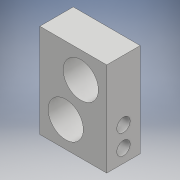
# Autodesk Inventor part: Part2
Saved by Autodesk Inventor 2017 (Build 210142000, 142)
## iProperties
Created: 2021-05-13
Part Number: Part2
Material: Generic
Document SubType Name: Modeling
Designer: majch
Density: 1 g/cm^3
Appearance: Default
Author: majch
Autodesk Inventor part; units mm, degrees
ref_plane "YZ Plane" through (0, 0, 0) normal (1, 0, 0) x (0, 1, 0)
ref_plane "XZ Plane" through (0, 0, 0) normal (0, 1, 0) x (-1, 0, 0)
ref_plane "XY Plane" through (0, 0, 0) normal (0, 0, 1) x (1, 0, 0)
sketch "Sketch1" plane through (0, 0, 0) normal (0, 1, 0) x (-1, 0, 0)
  line L0 (30, 18.75) -> (-10, 18.75)
  line L1 (30, 18.75) -> (30, -37.25)
  line L2 (-10, 18.75) -> (-10, -37.25)
  line L3 (-10, -37.25) -> (30, -37.25)
  circle A0 centre (5.5, 3.25) radius 10.5
  circle A1 centre (14.5, -21.75) radius 10.5
  point P0 (0, 0)
  dimension "szerokosc_jakas" = 40
  dimension "dlugosc_docisku" = 56
  dimension "srendica_walka" = 21
  dimension "odsuniecie_walka" = 15.5
  dimension "d4" = 15.5
  dimension "d5" = 21
  dimension "przesuniecie_wzgledne_walkow" = 9
  dimension "d7" = 25
  constraints: 8 end point, 2 centre point, 2 perpendicular, 1 horizontal
  measures "szerokosc_jakas" distance of L0.start L0.end
  measures "dlugosc_docisku" distance of L0.start L1.end
  measures "srendica_walka" diameter of A0
  measures "odsuniecie_walka" distance from line of L0 A0.centre
  measures "d4" distance from line of L2 A0.centre
  measures "d5" diameter of A1
  measures "przesuniecie_wzgledne_walkow" horizontal distance of A0.centre A1.centre
  measures "d7" vertical distance of A0.centre A1.centre
extrude "Extrusion1" add sketch "Sketch1" along normal blind 20
sketch "Sketch2" plane through (10, 0, 18.75) normal (1, 0, 0) x (0, 0, -1)
  circle A0 centre (48, 10) radius 4
  line L0 (56, 0) -> (56, 20) projected
  line L1 (0, 20) -> (56, 20) construction
  circle A1 centre (36, 10) radius 4
  line L2 (69, 10) -> (-3, 10) construction
  point P0 (18.75, 0)
  dimension "d10" = 8
  dimension "d11" = 8
  dimension "d15" = 12
  dimension "d25" = 10
  constraints: 2 centre point, 2 end point, 2 point on line, 1 horizontal
  measures "d10" diameter of A0
  measures "d11" distance from line of L0 A0.centre
  measures "d15" distance of A1.centre A0.centre
  measures "d25" distance between parallel lines of L1 L2
extrude "Extrusion2" cut sketch "Sketch2" against normal blind 10
sketch "Sketch3" plane through (-30, 0, -37.25) normal (-1, 0, 0) x (0, 0, 1)
  circle A0 centre (48, 10) radius 4
  circle A1 centre (36, 10) radius 4
  line L0 (56, 0) -> (56, 20) projected
  line L1 (0, 0) -> (56, 0) projected
  line L2 (75, 10) -> (-12, 10) construction
  point P0 (37.25, 0)
  dimension "d18" = 8
  dimension "d19" = 8
  dimension "d21" = 8
  dimension "d22" = 12
  dimension "d24" = 10
  constraints: 2 centre point, 2 end point, 2 point on line, 1 horizontal
  measures "d18" diameter of A0
  measures "d19" diameter of A1
  measures "d21" distance from line of L0 A0.centre
  measures "d22" distance of A1.centre A0.centre
  measures "d24" distance between parallel lines of L1 L2
extrude "Extrusion3" cut sketch "Sketch3" against normal blind 10
equation "\"szerokosc_jakas\" = szerokosc"
equation "\"dlugosc_docisku\" = dlugosc"
equation "\"srendica_walka\" = srednica_walka"
equation "\"d4\" = -0.5 * przesuniecie_wzgledne_walkow + 0.5 * szerokosc_jakas"
equation "\"d5\" = srednica_walka"
equation "\"d25\" = 0.5 * grubosc"
equation "\"gw\" = glebokosc_gwintu"
equation "\"d24\" = 0.5 * grubosc"
equation "\"d26\" = glebokosc_gwintu"
equation "\"glebokosc_gwintu\" = 10"
equation "\"szerokosc\" = 40"
equation "\"dlugosc\" = 56"
equation "\"srednica_walka\" = 21"
equation "\"grubosc\" = 20"
body "Solid1"
